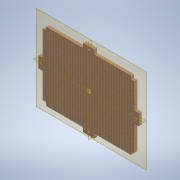
# Autodesk Inventor part: MDF_Base
Saved by Autodesk Inventor 2021 (Build 250183000, 183)
## iProperties
Created: 2021-02-17
Part Number: MDF_Base
Material: MDF Medium Density Fiberboard
Document SubType Name: Modeling
Designer: negt20
Density: 0.8 g/cm^3
Appearance: Cardboard - Corrugated
Author: negt20
Autodesk Inventor part; units mm, degrees
sketch "Sketch1" plane through (0, 0, 0) normal (0, 0, 1) x (1, 0, 0)
  line L0 (-99.5, 74.5) -> (99.5, 74.5)
  line L1 (99.5, 74.5) -> (99.5, -74.5)
  line L2 (99.5, -74.5) -> (-99.5, -74.5)
  line L3 (-99.5, -74.5) -> (-99.5, 74.5)
  point P0 (0, 74.5)
  point P1 (0, 0)
  point P2 (-99.5, 0)
  dimension "d0" = 199
  dimension "d1" = 149
  constraints: 8 end point, 2 midpoint, 2 parallel, 1 horizontal, 1 horizontal alignment, 1 perpendicular, 1 vertical alignment
  measures "d0" distance of L1.end L2.end
  measures "d1" distance of L0.end L1.end
extrude "Extrusion1" add sketch "Sketch1" along normal blind 6
sketch "Sketch2" plane through (0, 0, 6) normal (0, 0, 1) x (1, 0, 0)
  line L0 (-99.5, -74.5) -> (99.5, -74.5) projected
  line L1 (-99.5, -74.5) -> (-92.5, -74.5)
  line L2 (-92.5, -74.5) -> (-92.5, -67.5)
  line L3 (-92.5, -67.5) -> (-99.5, -67.5)
  line L4 (-99.5, -67.5) -> (-99.5, -74.5)
  point P0 (0, 0)
  point P1 (40.5, -62.5)
  dimension "d18" = 7
  dimension "d19" = 7
  constraints: 8 end point, 2 parallel, 1 horizontal, 1 perpendicular
  measures "d18" distance of L3.end L2.end
  measures "d19" distance of L2.end L1.end
extrude "Extrusion2" cut sketch "Sketch2" against normal blind 15
mirror "Mirror3" about plane through (0, 0, 0) normal (1, 0, 0) of "Extrusion2"
mirror "Mirror4" about plane through (0, 0, 0) normal (0, 1, 0) of "Extrusion2", "Mirror3"
sketch "Sketch4" plane through (0, 0, 6) normal (0, 0, 1) x (1, 0, 0)
  line L0 (-99.5, 67.5) -> (-99.5, -67.5) projected
  line L1 (-99.5, 12.5) -> (-109, 12.5)
  line L2 (-109, 12.5) -> (-109, -12.5)
  line L3 (-109, -12.5) -> (-99.5, -12.5)
  line L4 (-99.5, -12.5) -> (-99.5, 12.5)
  line L5 (-99.5, 0) -> (-103, 0) construction
  circle A0 centre (-103, 0) radius 2.1
  point P0 (0, 0)
  point P1 (-82, 49)
  point P2 (-82, -49)
  point P3 (-99.5, 0)
  point P4 (-99.5, -67.5)
  dimension "d23" = 9.5
  dimension "d24" = 25
  dimension "d34" = 3.5
  dimension "d35" = 4.2
  constraints: 10 end point, 2 coincident, 2 parallel, 1 centre point, 1 horizontal, 1 midpoint, 1 perpendicular, 3 other
  measures "d23" distance of L3.end L2.end
  measures "d24" distance between parallel lines of L3 L1
  measures "d34" distance of L5.start L5.end
  measures "d35" diameter of A0
extrude "Extrusion4" add sketch "Sketch4" against normal blind 6
mirror "Mirror5" about plane through (0, 0, 0) normal (1, 0, 0) of "Extrusion4"
sketch "Sketch6" plane through (0, 0, 6) normal (0, 0, 1) x (1, 0, 0)
  line L0 (92.5, 74.5) -> (-92.5, 74.5) projected
  line L1 (-12.5, 74.5) -> (12.5, 74.5)
  line L2 (12.5, 74.5) -> (12.5, 84)
  line L3 (12.5, 84) -> (-12.5, 84)
  line L4 (-12.5, 84) -> (-12.5, 74.5)
  circle A0 centre (0, 77.5) radius 2.1
  line L5 (0, 74.5) -> (0, 77.5) construction
  point P0 (0, 0)
  dimension "d28" = 25
  dimension "d29" = 9.5
  dimension "d30" = 4.2
  dimension "d36" = 3
  constraints: 10 end point, 2 coincident, 2 midpoint, 2 parallel, 1 centre point, 1 horizontal, 1 perpendicular, 1 point on line, 1 vertical
  measures "d28" distance of L3.end L2.end
  measures "d29" distance of L2.end L1.end
  measures "d30" diameter of A0
  measures "d36" distance of L5.start L5.end
extrude "Extrusion5" add sketch "Sketch6" against normal blind 6
mirror "Mirror6" about plane through (0, 0, 0) normal (0, 1, 0) of "Extrusion5"
fillet "Fillet4" radius 1 28 edges at (-109, -12.5, 3) (-99.5, -12.5, 3) (-99.5, -67.5, 3) (-92.5, -67.5, 3) (-92.5, -74.5, 3) (-12.5, -74.5, 3) (-12.5, -84, 3) (12.5, -84, 3) (92.5, -74.5, 3) (99.5, -67.5, 3) (12.5, -74.5, 3) (92.5, -67.5, 3) (99.5, -12.5, 3) (109, -12.5, 3) (109, 12.5, 3) (99.5, 67.5, 3) (92.5, 74.5, 3) (12.5, 84, 3) (92.5, 67.5, 3) (99.5, 12.5, 3) (-12.5, 84, 3) (-92.5, 74.5, 3) (-99.5, 67.5, 3) (-12.5, 74.5, 3) (-92.5, 67.5, 3) (-99.5, 12.5, 3) (-109, 12.5, 3) (12.5, 74.5, 3)
sketch "Sketch7" plane through (0, 0, 6) normal (0, 0, 1) x (1, 0, 0)
  circle A0 centre (0, 0) radius 8.25
  dimension "d38" = 16.5
  constraints: 1 centre point, 1 coincident
  measures "d38" diameter of A0
extrude "Extrusion6" cut sketch "Sketch7" against normal through all
equation "\"d7\" = d5"
equation "\"d5\" = 15"
body "Solid1"
